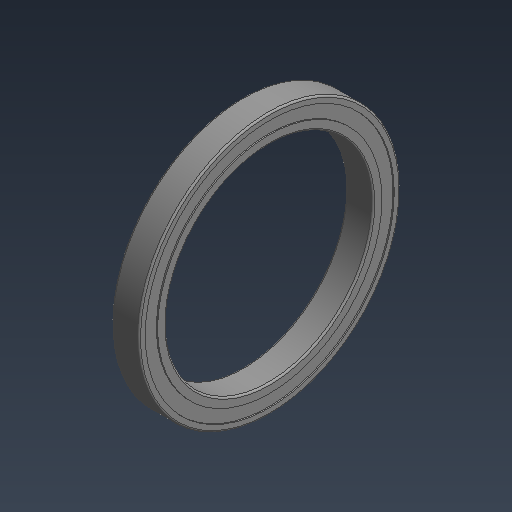
# Autodesk Inventor part: B6815ZZ
Saved by Autodesk Inventor 2021 (Build 250183000, 183)
## iProperties
Category: PARTsolutions
Company: MISUMI
Part Number: B6815ZZ
Material: 一般
Catalog Web Link: www.cadenas.de
Description: B6_ _ _ZZ, SB6_ _ _ZZ-Deep Groove Ball Bearings - Double Shield Type
Vendor: MISUMI
Document SubType Name: Modeling
Designer: partserver
Manufacturer: MISUMI
Mass: 25.5067 g
Surface Area: 109.028 cm^2
Volume: 25.5067 cm^3
Density: 1 g/cm^3
Appearance: PSOLRGB-175-175-175
PSOL_IDENT_0: {$CADENAS_DATA\23d-libs\misumi\metric\12_bearing_holders\sb6010zz.prj},172 {VTYP=3D},{NB=B6815ZZ},{L
PSOL_IDENT_1: INA=B6815ZZ},{NN=B6_ _ _ZZ, SB6_ _ _ZZ},{DATE=30.06.2021 12:59:24},{GEOMDATE=22.10.2019 06:26:04},{V
PSOL_IDENT_2: ERSION=},{LINEID=970},{WBVAR=TS},{WBNUMERIC=}  {NB=B6815ZZ},{LINA=B6815ZZ},{KT=DUMMY},{PN=B6815ZZ},{
PSOL_IDENT_3: TS=},{TS1= '', 'Steel'},{MAT=52100 Bearing Steel},{BN=6815ZZ},{DD=75},{D=95},{B=10},{RR=0.6},{CR=12.
PSOL_IDENT_4: 5},{COR=12.9},{CRS=12.5},{CRSS=-},{CORS=12.9},{CORSS=-},{DD1=0.00},{R1=0.00},{R2=0.0},{DSMIN=79.0},{
PSOL_IDENT_5: DSMAX=80.00},{DS1=80.00},{DDHH=91.0},{R=0.6},{MASS=145},{MASS11=145},{AA=9.0800},{BB=2.3111},{CC=3.2
PSOL_IDENT_6: 000},{TYS=w/o Retaining Ring}
NB: B6815ZZ
NN: B6_ _ _ZZ, SB6_ _ _ZZ
NT: Deep Groove Ball Bearings - Double Shield Type
NBSYN: $PN.
LINA: B6815ZZ
CATALOG: Misumi
PN: B6815ZZ
TS: Steel
MAT: 52100 Bearing Steel
BN: 6815ZZ
DD: 75
D: 95
B: 10
RR: 0.6
CR: 12.5
COR: 12.9
DSMIN: 79
DSMAX: 80
DDHH: 91
R: 0.6
MASS: 145
SUPPLIER: MISUMI
ARTICLENO: B6815ZZ
BOMINFO: B6815ZZ
CREATOR: CADENAS GmbH
購入先: ミスミ
在庫数: 0.0
Title: B6815ZZ
Author: Cadenas PARTsolutions
Comments: Deep Groove Ball Bearings - Double Shield Type
Autodesk Inventor part; units mm, degrees
sketch "Sketch_1" plane through (0, 0, 0) normal (0, 0, 1) x (1, 0, 0)
  line L0 (10, 0) -> (0, 0)
  arc A0 (0, 38.1) -> (0.6, 37.5) centre (0.6, 38.1) ccw
  line L1 (0.6, 37.5) -> (9.4, 37.5)
  arc A1 (9.4, 37.5) -> (10, 38.1) centre (9.4, 38.1) ccw
  line L2 (10, 38.1) -> (10, 40.7)
  line L3 (10, 40.7) -> (9.54, 40.7)
  line L4 (9.54, 40.7) -> (9.54, 45.1889)
  line L5 (9.54, 45.1889) -> (10, 45.1889)
  line L6 (10, 45.1889) -> (10, 46.9)
  arc A2 (10, 46.9) -> (9.4, 47.5) centre (9.4, 46.9) ccw
  line L7 (9.4, 47.5) -> (0.6, 47.5)
  arc A3 (0.6, 47.5) -> (0, 46.9) centre (0.6, 46.9) ccw
  line L8 (0, 46.9) -> (0, 45.1889)
  line L9 (0, 45.1889) -> (0.46, 45.1889)
  line L10 (0.46, 45.1889) -> (0.46, 40.7)
  line L11 (0.46, 40.7) -> (0, 40.7)
  line L12 (0, 40.7) -> (0, 38.1)
  constraints: 26 end point, 8 point on circle, 4 centre point
revolve "Revolution1" add sketch "Sketch_1" angle 360 about axis through (10, 0, 0) along (1, 0, 0)
ref_plane "center_point_XY" through (5, 0, 0) normal (1, 0, 0) x (0, 0, -1)
ref_plane "center_point_YZ" through (5, 0, 0) normal (0, 0, -1) x (0, 1, 0)
ref_plane "center_point_ZX" through (5, 0, 0) normal (0, 1, 0) x (1, 0, 0)
ref_plane "to_housing_XY" through (0, 0, 0) normal (1, 0, 0) x (0, 0, -1)
ref_plane "to_housing_YZ" through (0, 0, 0) normal (0, 0, -1) x (0, 1, 0)
ref_plane "to_housing_ZX" through (0, 0, 0) normal (0, 1, 0) x (1, 0, 0)
ref_plane "to_ring_XY" through (9.08, 0, 0) normal (1, 0, 0) x (0, 0, -1)
ref_plane "to_ring_YZ" through (9.08, 0, 0) normal (0, 0, -1) x (0, 1, 0)
ref_plane "to_ring_ZX" through (9.08, 0, 0) normal (0, 1, 0) x (1, 0, 0)
body "Solid1"
